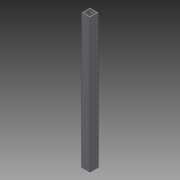
# Autodesk Inventor part: Part5
Saved by Autodesk Inventor 2015 (Build 190159000, 159)
## iProperties
Created: 2015-07-04
Part Number: Part5
Material: Generic
Document SubType Name: Modeling
Designer: tsayman
Density: 1 g/cm^3
Appearance: Default
Author: tsayman
Autodesk Inventor part; units mm, degrees
ref_plane "YZ Plane" through (0, 0, 0) normal (1, 0, 0) x (0, 1, 0)
ref_plane "XZ Plane" through (0, 0, 0) normal (0, 1, 0) x (-1, 0, 0)
ref_plane "XY Plane" through (0, 0, 0) normal (0, 0, 1) x (1, 0, 0)
sketch "Sketch1" plane through (0, 0, 0) normal (0, 0, 1) x (1, 0, 0)
  line L0 (-87.5495, -540.2269) -> (-62.1495, -540.2269)
  line L1 (-62.1495, -540.2269) -> (-62.1495, -946.6269)
  line L2 (-62.1495, -946.6269) -> (-87.5495, -946.6269)
  line L3 (-87.5495, -946.6269) -> (-87.5495, -540.2269)
  point P0 (0, 0)
  dimension "d0" = 25.4
  dimension "d1" = 406.4
  constraints: 8 end point, 2 parallel, 1 horizontal, 1 perpendicular
  measures "d0" distance of L1.end L2.end
  measures "d1" distance of L0.end L1.end
extrude "Extrusion1" add sketch "Sketch1" along normal blind 25.4
shell "Shell1" thickness 3.175 removed faces 2 at (-79.0829, -540.2269, 16.9333) at (-70.6162, -946.6269, 16.9333)
body "Solid1"
